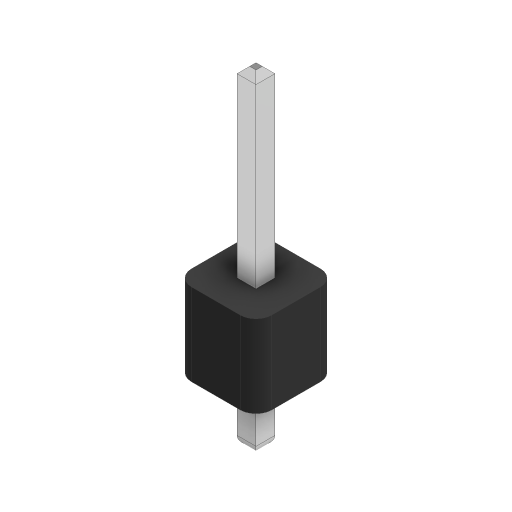
# Autodesk Inventor part: PIR pins
Saved by Autodesk Inventor 2024 (Build 280153000, 153)
## iProperties
Created: 2024-09-24
Part Number: PIR pins
Material: Generic
Document SubType Name: Modeling
Designer: Laith Al-Sadi
Density: 1 g/cm^3
Appearance: Default
Author: Laith Al-Sadi
Autodesk Inventor part; units mm, degrees
ref_plane "YZ Plane" through (0, 0, 0) normal (1, 0, 0) x (0, 1, 0)
ref_plane "XZ Plane" through (0, 0, 0) normal (0, 1, 0) x (-1, 0, 0)
ref_plane "XY Plane" through (0, 0, 0) normal (0, 0, 1) x (1, 0, 0)
sketch "Sketch1" plane through (0, 0, 0) normal (0, 1, 0) x (-1, 0, 0)
  line L0 (1.27, 1.27) -> (-1.27, 1.27)
  line L1 (-1.27, 1.27) -> (-1.27, -1.27)
  line L2 (-1.27, -1.27) -> (1.27, -1.27)
  line L3 (1.27, -1.27) -> (1.27, 1.27)
  line L4 (1.27, 1.27) -> (-1.27, -1.27) construction
  line L5 (-1.27, 1.27) -> (1.27, -1.27) construction
  point P0 (0, 0)
  dimension "d0" = 2.54
  dimension "d1" = 2.54
  constraints: 12 end point, 2 midpoint, 2 parallel, 1 horizontal, 1 perpendicular
  measures "d0" distance of L2.end L0.start
  measures "d1" distance of L1.end L2.end
extrude "Extrusion1" add sketch "Sketch1" along normal blind 2.6
fillet "Fillet1" radius 0.5 4 edges at (1.27, 1.3, 1.27) (1.27, 1.3, -1.27) (-1.27, 1.3, 1.27) (-1.27, 1.3, -1.27)
sketch "Sketch2" plane through (0, 2.6, 0) normal (0, 1, 0) x (1, 0, 0)
  line L0 (-0.3, -0.3) -> (0.3, -0.3)
  line L1 (0.3, -0.3) -> (0.3, 0.3)
  line L2 (0.3, 0.3) -> (-0.3, 0.3)
  line L3 (-0.3, 0.3) -> (-0.3, -0.3)
  line L4 (-0.3, -0.3) -> (0.3, 0.3) construction
  line L5 (0.3, -0.3) -> (-0.3, 0.3) construction
  point P0 (0, 0)
  dimension "d5" = 0.6
  dimension "d6" = 0.6
  constraints: 12 end point, 2 midpoint, 2 parallel, 1 horizontal, 1 perpendicular
  measures "d5" distance of L2.end L1.end
  measures "d6" distance of L1.end L0.end
extrude "Extrusion2" add sketch "Sketch2" along normal blind 5.8
chamfer "Chamfer1" distance 0.2 angle 45 4 edges at (0.3, 8.4, 0) (0, 8.4, 0.3) (-0.3, 8.4, 0) (0, 8.4, -0.3)
sketch "Sketch3" plane through (0, 0, 0) normal (0, -1, 0) x (1, 0, 0)
  line L0 (0.3, 0.3) -> (-0.3, 0.3) projected
  line L1 (-0.3, 0.3) -> (-0.3, -0.3) projected
  line L2 (-0.3, -0.3) -> (0.3, -0.3) projected
  line L3 (0.3, -0.3) -> (0.3, 0.3) projected
  point P0 (0, 0)
extrude "Extrusion3" add sketch "Sketch3" along normal blind 2
fillet "Fillet2" radius 0.28 4 edges at (0, -2, -0.3) (-0.3, -2, 0) (0, -2, 0.3) (0.3, -2, 0)
body "Solid1"
